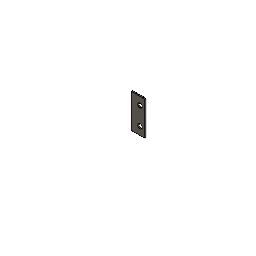
Spacer (Autodesk Fusion 360 design; units mm, degrees)
Autodesk Fusion 360 part; units mm, degrees
sketch "Sketch1" plane through (0, 0, 416.35) normal (0, 0, -1) x (-1, 0, 0)
  circle A0 centre (-237.4786, -269.9414) radius 1.6
  circle A1 centre (-237.4786, -256.5312) radius 1.6
  line L0 (-241.1286, -275.9414) -> (-228.1286, -275.9414)
  line L1 (-228.1286, -275.9414) -> (-228.1286, -250.5312)
  line L2 (-228.1286, -250.5312) -> (-241.1286, -250.5312)
  line L3 (-241.1286, -250.5312) -> (-241.1286, -275.9414)
  line L4 (-231.1286, -250.5312) -> (-231.1286, -275.9414)
extrude "Extrude1" add sketch "Sketch1" along normal blind 1 contours L0 L2 L3 L4
